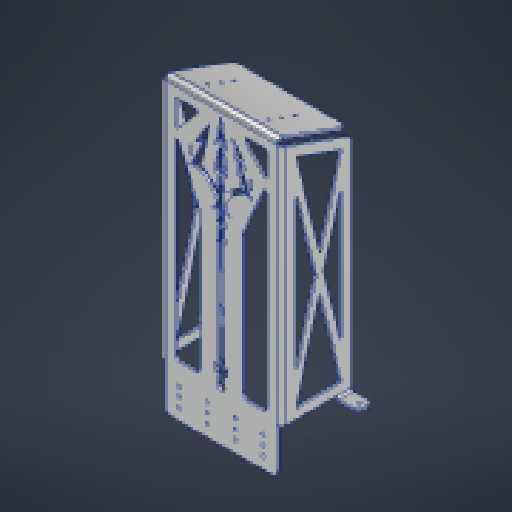
# Autodesk Inventor part: feeder_front_support
Saved by Autodesk Inventor 2024.3 (Build 283343010, 343A)
## iProperties
Created: 2025-03-08
Part Number: feeder_front_support
Material: Aluminum 6061
Document SubType Name: Sheet Metal
Designer: marcu
Density: 2.7 g/cm^3
Sheet Metal Rule: Default
Appearance: Aluminum - Flat
Flat Pattern Width: 34.4563 cm
Flat Pattern Length: 49.4576 cm
Flat Pattern Area: 1704.13 cm^2
Sheet Metal Width: 13.565 in
Sheet Metal Length: 19.472 in
Sheet Metal Area: 264.140 in^2
Mass: 692.047 g
Surface Area: 1786.85 cm^2
Volume: 256.314 cm^3
Author: marcu
Autodesk Inventor part; units mm, degrees
ref_plane "YZ Plane" through (0, 0, 0) normal (1, 0, 0) x (0, 1, 0)
ref_plane "XZ Plane" through (0, 0, 0) normal (0, 1, 0) x (-1, 0, 0)
ref_plane "XY Plane" through (0, 0, 0) normal (0, 0, 1) x (1, 0, 0)
sketch "Sketch20" plane through (0, 0, 0) normal (0, 0, 1) x (1, 0, 0)
  line L0 (-76.2, 201.168) -> (76.2, 201.168)
  line L1 (76.2, 201.168) -> (76.2, -201.168)
  line L2 (76.2, -201.168) -> (-76.2, -201.168)
  line L3 (-76.2, -201.168) -> (-76.2, 201.168)
  line L4 (-76.2, 201.168) -> (76.2, -201.168) construction
  line L5 (76.2, 201.168) -> (-76.2, -201.168) construction
  point P0 (0, 0)
  dimension "d149" = 152.4
  dimension "d150" = 402.336
  measures "d149" distance of L1.end L2.end
  measures "d150" distance of L0.end L1.end
extrude "Plate9" add sketch "Sketch20" along normal blind 3.175
sketch "Sketch21" plane through (76.2, 198.1845, 4.2609) normal (0, 0.9396926, -0.3420201) x (-1, 0, 0)
  line L0 (152.4, 0) -> (0, 0)
  line L1 (0, 0) -> (0, -101.6)
  line L2 (0, -101.6) -> (152.4, -101.6)
  line L3 (152.4, -101.6) -> (152.4, 0)
  constraints: 6 end point, 1 horizontal, 1 perpendicular, 1 vertical
edge flange "Flange6" height 101.6 angle 110 thickness 3.175 bend radius 3.175 thickness toward (0, 0.9396926, -0.3420201) relief straight relief width 3.175 relief depth 1.5875 edges at (0, 201.168, 0) wall of the first edge with corners at (-76.2, 198.1845, 4.2609) (76.2, 198.1845, 4.2609) (76.2, 163.4352, -91.2119) (-76.2, 163.4352, -91.2119)
bend "Bend7"
corner "Corner7"
sketch "Sketch22" plane through (0, 0, 3.175) normal (0, 0, 1) x (1, 0, 0)
  line L0 (76.2, -201.168) -> (-76.2, -201.168) projected
  line L1 (-76.2, -201.168) -> (-76.2, 192.0993) projected
  point P0 (0, 0)
  point P1 (-57.15, -185.293)
  point P2 (-57.15, -172.593)
  point P3 (-57.15, -159.893)
  point P4 (-44.45, -185.293)
  point P5 (-44.45, -172.593)
  point P6 (-44.45, -159.893)
  point P7 (-31.75, -185.293)
  point P8 (-31.75, -172.593)
  point P9 (-31.75, -159.893)
  point P10 (-19.05, -185.293)
  point P11 (-19.05, -172.593)
  point P12 (-19.05, -159.893)
  point P13 (-6.35, -185.293)
  point P14 (-6.35, -172.593)
  point P15 (-6.35, -159.893)
  point P16 (6.35, -185.293)
  point P17 (6.35, -172.593)
  point P18 (6.35, -159.893)
  point P19 (19.05, -185.293)
  point P20 (19.05, -172.593)
  point P21 (19.05, -159.893)
  point P22 (31.75, -185.293)
  point P23 (31.75, -172.593)
  point P24 (31.75, -159.893)
  point P25 (44.45, -185.293)
  point P26 (44.45, -172.593)
  point P27 (44.45, -159.893)
  point P28 (57.15, -185.293)
  point P29 (57.15, -172.593)
  point P30 (57.15, -159.893)
  dimension "d162" = 15.875
  dimension "d163" = 19.05
  dimension "d166" = 12.7
  dimension "d169" = 12.7
  constraints: 1 horizontal, 1 vertical, 29 other
  measures "d162" distance from line of L0 point (-57.15, -185.293)
  measures "d163" distance from line of L1 point (-57.15, -185.293)
  measures "d166" distance of point (-57.15, -185.293) point (-57.15, -172.593)
  measures "d169" distance of point (-57.15, -185.293) point (-44.45, -185.293)
hole "Hole5" at (-57.15, -185.293, 3.175) at (-57.15, -172.593, 3.175) at (-57.15, -159.893, 3.175) at (-19.05, -185.293, 3.175) at (-19.05, -159.893, 3.175) at (19.05, -185.293, 3.175) at (19.05, -159.893, 3.175) at (57.15, -185.293, 3.175) at (57.15, -172.593, 3.175) at (57.15, -159.893, 3.175) at (-19.05, -172.593, 3.175) at (19.05, -172.593, 3.175) direction (0, 0, -1) diameter 4.953 end through all clearance for "Flat Head Machine Screw (82)" size "#10" standard "Ansi Unified Screw Threads"
sketch "Sketch23" plane through (-79.375, 192.0993, -3.175) normal (-1, 0, 0) x (0, -1, 0)
  line L0 (393.2673, 0) -> (0, 0)
  line L1 (0, 0) -> (0, -88.9)
  line L2 (0, -88.9) -> (393.2673, -88.9)
  line L3 (393.2673, -88.9) -> (393.2673, 0)
  constraints: 6 end point, 1 horizontal, 1 perpendicular, 1 vertical
edge flange "Flange7" height 95.25 angle 90 thickness 3.175 bend radius 3.175 thickness toward (-1, 0, 0) relief straight relief width 3.175 relief depth 1.5875 edges at (-76.2, -4.5344, 0) wall of the first edge with corners at (-79.375, -201.168, -3.175) (-79.375, 192.0993, -3.175) (-79.375, 192.0993, -92.075) (-79.375, -201.168, -92.075)
bend "Bend8"
corner "Corner8"
sketch "Sketch24" plane through (79.375, -201.168, -3.175) normal (1, 0, 0) x (0, 1, 0)
  line L0 (393.2673, 0) -> (0, 0)
  line L1 (0, 0) -> (0, -88.9)
  line L2 (0, -88.9) -> (393.2673, -88.9)
  line L3 (393.2673, -88.9) -> (393.2673, 0)
  constraints: 6 end point, 1 horizontal, 1 perpendicular, 1 vertical
edge flange "Flange8" height 95.25 angle 90 thickness 3.175 bend radius 3.175 thickness toward (1, 0, 0) relief straight relief width 3.175 relief depth 1.5875 edges at (76.2, -4.5344, 0) wall of the first edge with corners at (79.375, 192.0993, -3.175) (79.375, -201.168, -3.175) (79.375, -201.168, -92.075) (79.375, 192.0993, -92.075)
bend "Bend9"
corner "Corner9"
sketch "Sketch25" plane through (82.55, -201.168, -92.075) normal (1, 0, 0) x (0, 0, -1)
  line L0 (-88.9, 393.2673) -> (-95.25, 393.2673) projected
  line L1 (-95.25, 393.2673) -> (0, 358.5991)
  line L2 (0, 0) -> (0, 393.2673) projected
  line L3 (0, 393.2673) -> (0, 358.5991)
  line L4 (-95.25, 393.2673) -> (0, 393.2673)
  line L5 (-95.25, 393.2673) -> (-95.25, 0) projected
  line L6 (0, 0) -> (-95.25, 0)
  line L7 (-95.25, 0) -> (-95.25, 61.9125)
  line L8 (-95.25, 61.9125) -> (0, 61.9125)
  line L9 (0, 61.9125) -> (0, 0)
  point P0 (-92.075, 201.168)
  dimension "d199" = 20
  dimension "d202" = 61.9125
  constraints: 14 end point, 2 parallel, 2 perpendicular, 2 point on line, 1 collinear, 1 horizontal
  measures "d199" angle of L4 L1
  measures "d202" distance of L6.end L7.end
extrude "Cut5" cut sketch "Sketch25" against normal blind 6.35 contours L4 L2 L1 L0 | L8 L2 L6 L5
mirror "Mirror4" about plane through (0, 0, 0) normal (1, 0, 0) of "Cut5"
sketch "Sketch26" plane through (-85.725, -142.4305, -3.175) normal (0, -1, 0) x (1, 0, 0)
  line L0 (0, -88.9) -> (0, 0)
  line L1 (0, 0) -> (-25.4, 0)
  line L2 (-25.4, 0) -> (-25.4, -88.9)
  line L3 (-25.4, -88.9) -> (0, -88.9)
  constraints: 6 end point, 1 horizontal, 1 perpendicular, 1 vertical
edge flange "Flange9" height 31.75 angle 90 thickness 3.175 bend radius 3.175 thickness toward (0, -1, 0) relief straight relief width 3.175 relief depth 1.5875 corner gap 3.175 corner form 0 edges at (-82.55, -139.2555, -47.625) (82.55, -139.2555, -47.625) wall of the first edge with corners at (-85.725, -142.4305, -92.075) (-85.725, -142.4305, -3.175) (-111.125, -142.4305, -3.175) (-111.125, -142.4305, -92.075)
bend "Bend10"
corner "Corner10"
sketch "Sketch27" plane through (111.125, -145.6055, -92.075) normal (1, 0, 0) x (0, 0, -1)
  line L0 (-88.9, 6.35) -> (-95.25, 6.35) projected
  line L1 (0, 0) -> (-88.9, 0) projected
  line L2 (-88.9, 6.35) -> (-19.05, 6.35)
  line L3 (-19.05, 6.35) -> (-19.05, 0)
  line L4 (-19.05, 0) -> (-88.9, 0)
  line L5 (-88.9, 0) -> (-88.9, 6.35)
  point P0 (-92.075, 145.6055)
  dimension "d213" = 69.85
  constraints: 8 end point, 2 parallel, 1 horizontal, 1 perpendicular, 1 point on line
  measures "d213" distance of L0.start L2.end
extrude "Cut6" cut sketch "Sketch27" against normal blind 234.95
fillet "Corner Round3" radius 6.35 4 edges at (-111.125, -144.018, -73.025) (-111.125, -144.018, -92.075) (111.125, -144.018, -73.025) (111.125, -144.018, -92.075)
sketch "Sketch28" plane through (-85.725, -142.4305, -73.025) normal (0, 1, 0) x (1, 0, 0)
  line L0 (-19.05, 19.05) -> (0, 19.05) projected
  line L1 (-19.05, 0) -> (0, 0) projected
  line L2 (-25.4, 12.7) -> (-25.4, 6.35) projected
  line L3 (196.85, 6.35) -> (196.85, 12.7) projected
  point P0 (85.725, -73.025)
  point P1 (-17.4625, 9.525)
  point P2 (188.9125, 9.525)
  dimension "d217" = 9.525
  dimension "d218" = 19.05
  dimension "d219" = 7.9375
  dimension "d220" = 7.9375
  constraints: 1 horizontal alignment
  measures "d217" distance from line of L0 point (-17.462, 9.525)
  measures "d218" distance between parallel lines of L1 L0
  measures "d219" distance from line of L2 point (-17.462, 9.525)
  measures "d220" distance from line of point (188.912, 9.525) L3
hole "Hole6" at (-103.1875, -142.4305, -82.55) at (103.1875, -142.4305, -82.55) direction (0, -1, 0) diameter 4.953 end through all clearance for "Flat Head Machine Screw (82)" size "#10" standard "Ansi Unified Screw Threads"
sketch "Sketch29" plane through (0, 0, 3.175) normal (0, 0, 1) x (1, 0, 0)
  line L0 (-69.85, -137.668) -> (69.85, -137.668) construction
  line L1 (-69.85, -144.018) -> (69.85, -144.018)
  line L2 (69.85, -131.318) -> (-69.85, -131.318)
  arc A0 (-69.85, -131.318) -> (-69.85, -144.018) centre (-69.85, -137.668) ccw
  arc A1 (69.85, -144.018) -> (69.85, -131.318) centre (69.85, -137.668) ccw
  line L3 (-69.85, 185.7493) -> (69.85, 185.7493) construction
  line L4 (-69.85, 179.3993) -> (69.85, 179.3993)
  line L5 (69.85, 192.0993) -> (-69.85, 192.0993)
  arc A2 (-69.85, 192.0993) -> (-69.85, 179.3993) centre (-69.85, 185.7493) ccw
  arc A3 (69.85, 179.3993) -> (69.85, 192.0993) centre (69.85, 185.7493) ccw
  line L6 (-69.85, 185.7493) -> (-69.85, -137.668) construction
  line L7 (-76.2, 185.7493) -> (-76.2, -137.668)
  line L8 (-63.5, -137.668) -> (-63.5, 185.7493)
  arc A4 (-63.5, 185.7493) -> (-76.2, 185.7493) centre (-69.85, 185.7493) ccw
  arc A5 (-76.2, -137.668) -> (-63.5, -137.668) centre (-69.85, -137.668) ccw
  line L9 (69.85, -137.668) -> (69.85, 185.7493) construction
  line L10 (76.2, -137.668) -> (76.2, 185.7493)
  line L11 (63.5, 185.7493) -> (63.5, -137.668)
  arc A6 (63.5, -137.668) -> (76.2, -137.668) centre (69.85, -137.668) ccw
  arc A7 (76.2, 185.7493) -> (63.5, 185.7493) centre (69.85, 185.7493) ccw
  line L12 (76.2, 192.0993) -> (-76.2, 192.0993) projected
  line L13 (-76.2, -139.2555) -> (-76.2, 192.0993) projected
  line L14 (76.2, 192.0993) -> (76.2, -139.2555) projected
  line L15 (76.2, -201.168) -> (-76.2, -201.168) projected
  line L16 (69.85, 185.7493) -> (-69.85, -137.668) construction
  line L17 (65.4779, 187.6378) -> (-74.2221, -135.7795)
  line L18 (-65.4779, -139.5565) -> (74.2221, 183.8607)
  arc A8 (74.2221, 183.8607) -> (65.4779, 187.6378) centre (69.85, 185.7493) ccw
  arc A9 (-74.2221, -135.7795) -> (-65.4779, -139.5565) centre (-69.85, -137.668) ccw
  line L19 (-69.85, 185.7493) -> (69.85, -137.668) construction
  line L20 (-74.2221, 183.8607) -> (65.4779, -139.5565)
  line L21 (74.2221, -135.7795) -> (-65.4779, 187.6378)
  arc A10 (-65.4779, 187.6378) -> (-74.2221, 183.8607) centre (-69.85, 185.7493) ccw
  arc A11 (65.4779, -139.5565) -> (74.2221, -135.7795) centre (69.85, -137.668) ccw
  line L22 (-28.575, 179.3993) -> (28.575, 179.3993)
  line L23 (28.575, 179.3993) -> (28.575, -131.318)
  line L24 (28.575, -131.318) -> (-28.575, -131.318)
  line L25 (-28.575, -131.318) -> (-28.575, 179.3993)
  line L26 (-63.5, 143.0247) -> (-28.575, 62.1704)
  line L27 (63.5, 143.0247) -> (28.575, 62.1704)
  line L28 (-28.575, -30.1027) -> (-28.575, -54.1231)
  line L29 (-63.5, -110.957) -> (-63.5, -131.318)
  line L30 (-61.9193, -131.318) -> (-63.5, -131.318)
  line L31 (28.575, -30.1027) -> (28.575, -54.1231)
  line L32 (63.5, -110.957) -> (63.5, -131.318)
  line L33 (61.9193, -131.318) -> (63.5, -131.318)
  point P0 (0, 0)
  point P1 (0, -137.668)
  point P2 (0, 185.7493)
  point P3 (-69.85, 24.0406)
  point P4 (69.85, 24.0406)
  point P5 (0, 24.0406)
  point P6 (0, 24.0406)
  point P7 (5.1878, 24.0406)
  point P8 (63.5, 159.0383)
  point P9 (63.5, -134.9774)
  point P10 (0, 12.0304)
  point P11 (-63.5, -134.9774)
  point P12 (-5.1878, 24.0406)
  point P13 (-63.5, 159.0383)
  point P14 (-63.5, 183.0587)
  point P15 (0, 36.0508)
  point P16 (63.5, 183.0587)
  point P17 (63.5, 179.3993)
  point P18 (-63.5, 179.3993)
  point P19 (-72.5566, -131.9237)
  point P20 (72.5566, -131.9237)
  point P21 (61.9193, -131.318)
  point P22 (72.5566, 180.005)
  point P23 (-72.5566, 180.005)
  point P24 (76.2, 185.7493)
  point P25 (-61.9193, 179.3993)
  point P26 (61.9193, 179.3993)
  point P27 (0, -131.318)
  point P28 (28.575, 78.184)
  point P29 (-28.575, 78.184)
  point P30 (-28.575, -131.318)
  point P31 (-28.575, -54.1231)
  dimension "d228" = 12.7
  dimension "d229" = 12.7
  dimension "d230" = 12.7
  dimension "d231" = 12.7
  dimension "d232" = 57.15
  dimension "d233" = 9.525
  dimension "d234" = 9.525
  dimension "d250" = 28.575
  dimension "d251" = 28.575
  dimension "d252" = 6.35
  dimension "d253" = 6.35
  constraints: 72 end point, 28 tangent, 26 point on line, 24 point on circle, 12 centre point, 11 parallel, 7 midpoint, 3 perpendicular, 2 horizontal, 1 collinear, 1 concentric
  measures "d228" diameter of A1
  measures "d229" diameter of A3
  measures "d230" diameter of A5
  measures "d231" diameter of A7
  measures "d232" distance between parallel lines of L15 L1
  measures "d233" diameter of A9
  measures "d234" diameter of A11
  measures "d250" distance from line of point (0, -137.668) L23
  measures "d251" distance from line of L25 point (0, -131.318)
  measures "d252" distance between parallel lines of L20 L26
  measures "d253" distance between parallel lines of L18 L27
extrude "Extrusion3" cut sketch "Sketch29" against normal up to surface (3.175 mm away) contours L17 L25 L18 L2 L8 | L8 L26 L25 L17 | L18 L25 L2 | L21 L23 L27 L11 | L11 L2 L20 L23 L21 | L2 L23 L20
sketch "Sketch30" plane through (-82.55, -139.2555, -3.175) normal (-1, 0, 0) x (0, 0, 1)
  line L0 (-82.55, 292.2403) -> (-6.35, 319.9748) construction
  line L1 (-80.3782, 286.2732) -> (-4.1782, 314.0078)
  line L2 (-8.5218, 325.9419) -> (-84.7218, 298.2073)
  arc A0 (-84.7218, 298.2073) -> (-80.3782, 286.2732) centre (-82.55, 292.2403) ccw
  arc A1 (-4.1782, 314.0078) -> (-8.5218, 325.9419) centre (-6.35, 319.9748) ccw
  line L3 (-82.55, 6.35) -> (-6.35, 6.35) construction
  line L4 (-82.55, 0) -> (-6.35, 0)
  line L5 (-6.35, 12.7) -> (-82.55, 12.7)
  arc A2 (-82.55, 12.7) -> (-82.55, 0) centre (-82.55, 6.35) ccw
  arc A3 (-6.35, 0) -> (-6.35, 12.7) centre (-6.35, 6.35) ccw
  line L6 (-88.9, 0) -> (-88.9, 296.6866) projected
  line L7 (0, 0) -> (0, 329.0435) projected
  line L8 (-69.85, 0) -> (0, 0) projected
  line L9 (0, 329.0435) -> (-88.9, 296.6866) projected
  line L10 (-82.55, 6.35) -> (-82.55, 292.2403) construction
  line L11 (-76.2, 6.35) -> (-76.2, 292.2403)
  line L12 (-88.9, 292.2403) -> (-88.9, 6.35)
  arc A4 (-88.9, 6.35) -> (-76.2, 6.35) centre (-82.55, 6.35) ccw
  arc A5 (-76.2, 292.2403) -> (-88.9, 292.2403) centre (-82.55, 292.2403) ccw
  line L13 (-6.35, 6.35) -> (-6.35, 319.9748) construction
  line L14 (0, 6.35) -> (0, 319.9748)
  line L15 (-12.7, 319.9748) -> (-12.7, 6.35)
  arc A6 (-12.7, 6.35) -> (0, 6.35) centre (-6.35, 6.35) ccw
  arc A7 (0, 319.9748) -> (-12.7, 319.9748) centre (-6.35, 319.9748) ccw
  line L16 (-88.9, 0) -> (-69.85, 0) projected
  line L17 (-82.55, 292.2403) -> (-6.35, 6.35) construction
  line L18 (-87.1518, 291.0137) -> (-10.9518, 5.1234)
  line L19 (-1.7482, 7.5766) -> (-77.9482, 293.4668)
  arc A8 (-77.9482, 293.4668) -> (-87.1518, 291.0137) centre (-82.55, 292.2403) ccw
  arc A9 (-10.9518, 5.1234) -> (-1.7482, 7.5766) centre (-6.35, 6.35) ccw
  line L20 (-6.35, 319.9748) -> (-82.55, 6.35) construction
  line L21 (-10.9779, 321.0992) -> (-87.1779, 7.4744)
  line L22 (-77.9221, 5.2256) -> (-1.7221, 318.8504)
  arc A10 (-1.7221, 318.8504) -> (-10.9779, 321.0992) centre (-6.35, 319.9748) ccw
  arc A11 (-87.1779, 7.4744) -> (-77.9221, 5.2256) centre (-82.55, 6.35) ccw
  point P0 (3.175, 139.2555)
  point P1 (-44.45, 306.1075)
  point P2 (-44.45, 6.35)
  point P3 (-82.55, 149.2951)
  point P4 (-6.35, 163.1624)
  point P5 (-44.45, 149.2951)
  point P6 (-44.45, 163.1624)
  point P7 (-76.2, 52.6572)
  point P8 (-51.1268, 155.8536)
  point P9 (-76.2, 249.9241)
  point P10 (-45.9991, 136.615)
  point P11 (-76.1061, 12.7)
  point P12 (-12.9713, 12.7)
  point P13 (-12.7, 273.6676)
  point P14 (-41.2983, 155.9624)
  point P15 (-12.7, 48.6661)
  point P16 (-46.4261, 175.201)
  point P17 (-13.5276, 310.6048)
  point P18 (-76.2, 287.794)
  point P19 (-76.2, 286.908)
  dimension "d237" = 12.7
  dimension "d238" = 12.7
  dimension "d239" = 12.7
  dimension "d240" = 12.7
  dimension "d241" = 9.525
  dimension "d242" = 9.525
  constraints: 48 end point, 37 tangent, 24 point on circle, 12 centre point, 7 parallel, 6 midpoint, 1 horizontal, 1 perpendicular
  measures "d237" diameter of A1
  measures "d238" diameter of A3
  measures "d239" diameter of A5
  measures "d240" diameter of A7
  measures "d241" diameter of A9
  measures "d242" diameter of A11
extrude "Extrusion4" cut sketch "Sketch30" against normal blind 193.675 contours L1 L21 L19 L11 | L18 L21 L11 | L22 L15 L19 | L18 L5 L22
fillet "Corner Round4" radius 6.35 6 edges at (-80.9625, 157.4311, -92.075) (80.9625, 157.4311, -92.075) (-76.2, 164.927, -91.7548) (76.2, 164.927, -91.7548) (-76.2, -201.168, 1.5875) (76.2, -201.168, 1.5875)
fillet "Corner Round4" radius 1.5875 26 edges at (-80.9625, 148.5385, -79.375) (-80.9625, 147.6525, -79.375) (-80.9625, 110.6686, -79.375) (-80.9625, 134.4121, -15.875) (-80.9625, 35.9455, -49.6011) (-80.9625, 171.3493, -16.7026) (-80.9625, 16.7069, -44.4733) (-80.9625, 16.5981, -54.3018) (-80.9625, -86.5983, -79.375) (-80.9625, -90.5894, -15.875) (-80.9625, -126.5555, -16.1463) (-80.9625, -126.5555, -79.2811) (-80.9625, -2.6405, -49.1741) (80.9625, 171.3493, -16.7026) (80.9625, 148.5385, -79.375) (80.9625, 147.6525, -79.375) (80.9625, 35.9455, -49.6011) (80.9625, 110.6686, -79.375) (80.9625, 134.4121, -15.875) (80.9625, 16.7069, -44.4733) (80.9625, 16.5981, -54.3018) (80.9625, -86.5983, -79.375) (80.9625, -90.5894, -15.875) (80.9625, -2.6405, -49.1741) (80.9625, -126.5555, -16.1463) (80.9625, -126.5555, -79.2811)
sketch "Sketch32" plane through (0, 0, 3.175) normal (0, 0, 1) x (1, 0, 0)
  line L0 (-3.7084, 37.5903) -> (-3.7084, -98.2678)
  line L1 (34.204, 140.4917) -> (24.2324, 147.4624)
  arc A0 (-5.8261, 38.3768) -> (-3.7084, 37.5903) centre (0, 50.8205) ccw
  line L2 (36.8872, 111.2125) -> (27.5052, 109.2509)
  line L3 (-3.9118, 55.0386) -> (-5.8261, 38.3768)
  line L4 (7.8057, 150.3041) -> (0, 187.0662)
  line L5 (-1.8542, 55.6581) -> (-3.9118, 55.0386)
  line L6 (26.1652, 120.4316) -> (15.2743, 170.3618)
  arc A1 (-6.5188, 59.0194) -> (-1.8542, 55.6581) centre (0, 63.1484) ccw
  arc A2 (34.204, 140.4917) -> (15.2743, 170.3618) centre (-53.7033, 105.7152) ccw
  arc A3 (-6.5188, 59.0194) -> (-4.1604, 76.3719) centre (-39.8623, 72.3877) ccw
  arc A4 (4.6355, -117.0332) -> (9.0802, -107.1771) centre (-8.891, -105.0031) ccw
  line L7 (-1.8542, 79.1795) -> (-4.1604, 76.3719)
  arc A5 (4.1604, 76.3719) -> (6.5188, 59.0194) centre (39.8623, 72.3877) ccw
  line L8 (-1.8542, 81.235) -> (-1.8542, 79.1795)
  line L9 (3.9118, 55.0386) -> (5.8261, 38.3768)
  arc A6 (-13.1346, 73.4139) -> (-1.8542, 81.235) centre (-14.7446, 87.7815) ccw
  arc A7 (0, -137.002) -> (5.4561, -130.603) centre (-2.1439, -129.6484) ccw
  arc A8 (-13.1346, 73.4139) -> (-5.0523, 85.4275) centre (-26.1926, 90.9244) ccw
  line L10 (3.7084, -110.337) -> (9.0802, -107.1771)
  line L11 (3.7084, -121.0502) -> (8.4094, -115.5653)
  arc A9 (-5.0523, 85.4275) -> (-27.5052, 109.2509) centre (-60.3995, 55.7566) ccw
  line L12 (1.8542, 79.1795) -> (4.1604, 76.3719)
  line L13 (-3.7084, -121.0502) -> (-8.4094, -115.5653)
  line L14 (-36.8872, 111.2125) -> (-27.5052, 109.2509)
  arc A10 (3.7084, -103.8304) -> (3.7084, -98.2678) centre (0, -101.0491) ccw
  line L15 (4.8736, 100.0762) -> (25.0364, 115.6556)
  line L16 (-43.3723, 109.8571) -> (-36.8872, 111.2125)
  line L17 (3.7084, -103.8304) -> (3.7084, -110.337)
  arc A11 (27.5052, 109.2509) -> (5.0523, 85.4275) centre (60.3995, 55.7566) ccw
  line L18 (-38.8725, 114.4031) -> (-43.3723, 109.8571)
  line L19 (1.8542, 81.235) -> (1.8542, 79.1795)
  line L20 (4.8515, 143.1818) -> (8.5615, 118.0141)
  line L21 (-24.2324, 147.4624) -> (-38.8725, 114.4031)
  line L22 (3.7084, -121.0502) -> (3.7084, -127.8243)
  arc A12 (5.0523, 85.4275) -> (13.1346, 73.4139) centre (26.1926, 90.9244) ccw
  line L23 (-34.204, 140.4917) -> (-24.2324, 147.4624)
  line L24 (5.4561, -130.603) -> (3.7084, -127.8243)
  line L25 (-1.8542, 148.5435) -> (-4.8515, 143.1818)
  arc A13 (1.8542, 81.235) -> (13.1346, 73.4139) centre (14.7446, 87.7815) ccw
  line L26 (-7.8057, 150.3041) -> (-1.8542, 158.0065)
  line L27 (-4.8515, 143.1818) -> (-8.5615, 118.0141)
  line L28 (8.5615, 118.0141) -> (1.8542, 126.6945)
  line L29 (1.8542, 55.6581) -> (3.9118, 55.0386)
  line L30 (-7.8057, 150.3041) -> (0, 187.0662)
  line L31 (1.8542, 158.0065) -> (1.8542, 148.5435)
  line L32 (8.4094, -115.5653) -> (4.6355, -117.0332)
  arc A14 (-5.4561, -130.603) -> (0, -137.002) centre (2.1439, -129.6484) ccw
  line L33 (-3.7084, -121.0502) -> (-3.7084, -127.8243)
  line L34 (-3.7084, -103.8304) -> (-3.7084, -110.337)
  line L35 (3.7084, 37.5903) -> (3.7084, -98.2678)
  arc A15 (-3.7084, -98.2678) -> (-3.7084, -103.8304) centre (0, -101.0491) ccw
  line L36 (4.8736, 100.0762) -> (1.8542, 126.6945)
  line L37 (-3.7084, -110.337) -> (-9.0802, -107.1771)
  arc A16 (-9.0802, -107.1771) -> (-4.6355, -117.0332) centre (8.891, -105.0031) ccw
  line L38 (-5.4561, -130.603) -> (-3.7084, -127.8243)
  line L39 (-8.4094, -115.5653) -> (-4.6355, -117.0332)
  line L40 (-8.5615, 118.0141) -> (-1.8542, 126.6945)
  line L41 (38.8725, 114.4031) -> (43.3723, 109.8571)
  line L42 (-1.8542, 158.0065) -> (-1.8542, 148.5435)
  line L43 (25.0364, 115.6556) -> (30.0989, 114.4946)
  line L44 (-4.8736, 100.0762) -> (-1.8542, 126.6945)
  line L45 (43.3723, 109.8571) -> (36.8872, 111.2125)
  line L46 (-4.8736, 100.0762) -> (-25.0364, 115.6556)
  line L47 (1.8542, 148.5435) -> (4.8515, 143.1818)
  line L48 (-25.0364, 115.6556) -> (-30.0989, 114.4946)
  line L49 (7.8057, 150.3041) -> (1.8542, 158.0065)
  line L50 (-30.0989, 114.4946) -> (-26.1652, 120.4316)
  arc A17 (3.7084, 37.5903) -> (5.8261, 38.3768) centre (0, 50.8205) ccw
  line L51 (24.2324, 147.4624) -> (38.8725, 114.4031)
  line L52 (-26.1652, 120.4316) -> (-15.2743, 170.3618)
  line L53 (30.0989, 114.4946) -> (26.1652, 120.4316)
  arc A18 (-15.2743, 170.3618) -> (-34.204, 140.4917) centre (53.7033, 105.7152) ccw
  arc A19 (1.8542, 55.6581) -> (6.5188, 59.0194) centre (0, 63.1484) ccw
  point P0 (0, 0)
  point P1 (-6.5188, 59.0194)
  point P2 (-5.8261, 38.3768)
  point P3 (-4.6355, -117.0332)
  point P4 (-5.4561, -130.603)
  point P5 (0, -137.002)
  point P6 (5.4561, -130.603)
  point P7 (4.6355, -117.0332)
  point P8 (9.0802, -107.1771)
  point P9 (3.7084, -103.8304)
  point P10 (3.7084, -98.2678)
  point P11 (6.5188, 59.0194)
  point P12 (4.1604, 76.3719)
  point P13 (13.1346, 73.4139)
  point P14 (5.0523, 85.4275)
  point P15 (-27.5052, 109.2509)
  point P16 (-5.0523, 85.4275)
  point P17 (-4.1604, 76.3719)
  constraints: 108 end point, 40 point on circle, 20 centre point
extrude "Extrusion5" cut sketch "Sketch32" against normal blind 3.175
fillet "Corner Round5" radius 6.35 6 edges at (-28.575, 62.1704, 1.5875) (28.575, 62.1704, 1.5875) (28.575, -131.318, 1.5875) (63.5, -131.318, 1.5875) (-63.5, -131.318, 1.5875) (-28.575, -131.318, 1.5875)
fillet "Corner Round5" radius 3.175 2 edges at (-63.5, 143.0247, 1.5875) (63.5, 143.0247, 1.5875)
sketch "Sketch33" plane through (0, 0, 3.175) normal (0, 0, 1) x (1, 0, 0)
  line L0 (76.2, 192.0993) -> (-76.2, 192.0993) projected
  line L1 (-63.5, 127.6675) -> (-63.5, -124.968) projected
  line L2 (-76.2, 192.0993) -> (-63.5, 192.0993)
  line L3 (-63.5, 192.0993) -> (-63.5, 127.6675)
  line L4 (-63.5, 127.6675) -> (-76.2, 127.6675)
  line L5 (-76.2, 127.6675) -> (-76.2, 192.0993)
  line L6 (76.2, 192.0993) -> (76.2, -139.2555) projected
  line L7 (-76.2, 192.0993) -> (76.2, 192.0993)
  line L8 (76.2, 192.0993) -> (76.2, 179.3993)
  line L9 (76.2, 179.3993) -> (-76.2, 179.3993)
  line L10 (-76.2, 179.3993) -> (-76.2, 192.0993)
  line L11 (63.5, 127.6675) -> (63.5, -124.968) projected
  line L12 (76.2, 192.0993) -> (63.5, 192.0993)
  line L13 (63.5, 192.0993) -> (63.5, 127.6675)
  line L14 (63.5, 127.6675) -> (76.2, 127.6675)
  line L15 (76.2, 127.6675) -> (76.2, 192.0993)
  line L16 (-63.5, 138.1243) -> (-28.575, 179.3993)
  line L17 (28.575, 179.3993) -> (63.5, 138.1243)
  point P0 (0, 0)
  point P1 (63.5, 179.3993)
  point P2 (-63.5, 179.3993)
  dimension "d256" = 12.7
  dimension "d257" = 12.7
  dimension "d258" = 34.925
  dimension "d259" = 41.275
  dimension "d260" = 34.925
  constraints: 28 end point, 6 parallel, 5 point on line, 3 horizontal, 3 perpendicular, 1 equal length
  measures "d256" distance of L7.end L8.end
  measures "d257" distance of L14.end L11.start
  measures "d258" distance from line of L3 L16.end
  measures "d259" distance from line of L9 L16.start
  measures "d260" distance from line of L13 L17.start
extrude "Extrusion6" cut sketch "Sketch33" against normal up to surface (3.175 mm away) contours L13 L17 L9 | L9 L16 L3
fillet "Corner Round6" radius 3.175 6 edges at (-63.5, 179.3993, 1.5875) (-63.5, 138.1243, 1.5875) (-28.575, 179.3993, 1.5875) (28.575, 179.3993, 1.5875) (63.5, 138.1243, 1.5875) (63.5, 179.3993, 1.5875)
sketch "Sketch34" plane through (-76.2, 198.0663, -5.3468) normal (0, 0.9396926, -0.3420201) x (1, 0, 0)
  circle A0 centre (34.925, 16.2204) radius 2.6845 projected
  circle A1 centre (34.925, 35.2704) radius 2.6845 projected
  circle A2 centre (34.925, 54.3204) radius 2.6845 projected
  circle A3 centre (117.475, 35.2704) radius 2.6845 projected
  circle A4 centre (117.475, 54.3204) radius 2.6845 projected
  circle A5 centre (117.475, 16.2204) radius 2.6845 projected
  point P0 (76.2, 62.7183)
  point P1 (111.125, 51.6359)
  constraints: 4 other
hole "Hole7" at (41.275, 179.4876, -56.3913) at (41.275, 186.0031, -38.4902) at (41.275, 192.5186, -20.5891) at (-41.275, 192.5186, -20.5891) at (-41.275, 186.0031, -38.4902) at (-41.275, 179.4876, -56.3913) direction (0, -0.9396926, 0.3420201) diameter 4.5 depth 3.175 tip angle 118
equation "\"d151\" = Thickness"
equation "\"d152\" = BendReliefWidth"
equation "\"d153\" = BendReliefDepth"
equation "\"d154\" = MinimumRemnant"
equation "\"d155\" = TransitionRadius"
equation "\"d158\" = BendRadius"
equation "\"d159\" = CornerReliefSize"
equation "\"d160\" = GapSize"
equation "\"d161\" = JacobiRadiusSize"
equation "\"BendRadius\" = Thickness"
equation "\"BendReliefWidth\" = Thickness"
equation "\"BendReliefDepth\" = 0.5 * Thickness"
equation "\"CornerReliefSize\" = 4 * Thickness"
equation "\"MinimumRemnant\" = 2 * Thickness"
equation "\"TransitionRadius\" = BendRadius"
equation "\"JacobiRadiusSize\" = BendRadius"
equation "\"GapSize\" = Thickness"
equation "\"Thickness\" = 3.175"
body "Solid3"
